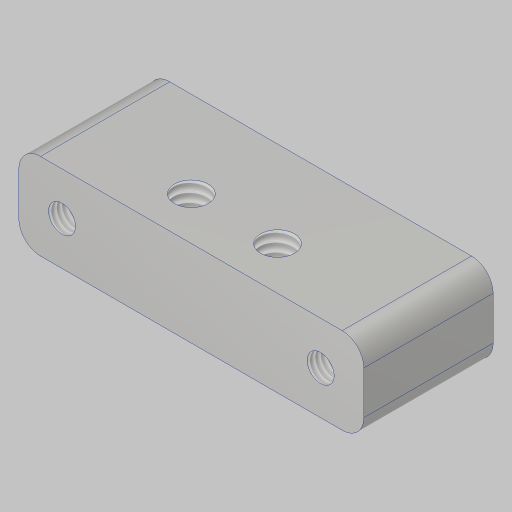
# Autodesk Inventor part: CL7-014
Saved by Autodesk Inventor 2023.5 (Build 275446000, 446)
## iProperties
Created: 2025-03-18
Part Number: CL7-014
Material: Aluminum 6061
Document SubType Name: Modeling
Designer: slick
Density: 2.7 g/cm^3
Appearance: Aluminum - Flat
Author: slick
Autodesk Inventor part; units mm, degrees
ref_plane "YZ Plane" through (0, 0, 0) normal (1, 0, 0) x (0, 1, 0)
ref_plane "XZ Plane" through (0, 0, 0) normal (0, 1, 0) x (-1, 0, 0)
ref_plane "XY Plane" through (0, 0, 0) normal (0, 0, 1) x (1, 0, 0)
sketch "Sketch1" plane through (0, 0, 0) normal (0, 0, 1) x (1, 0, 0)
  line L0 (25.4, -6.35) -> (-25.4, -6.35)
  line L1 (-25.4, -6.35) -> (-25.4, 6.35)
  line L2 (-25.4, 6.35) -> (25.4, 6.35)
  line L3 (25.4, 6.35) -> (25.4, -6.35)
  line L4 (25.4, -6.35) -> (-25.4, 6.35) construction
  line L5 (-25.4, -6.35) -> (25.4, 6.35) construction
  point P0 (0, 0)
  dimension "d0" = 50.8
  dimension "d1" = 12.7
  constraints: 12 end point, 2 midpoint, 2 parallel, 1 horizontal, 1 perpendicular
  measures "d0" distance of L1.end L2.end
  measures "d1" distance of L0.end L1.end
extrude "Extrusion1" add sketch "Sketch1" along normal blind 19.05
sketch "Sketch2" plane through (-25.4, 6.35, 0) normal (0, 1, 0) x (1, 0, 0)
  line L0 (0, 0) -> (0, -19.05) construction
  line L1 (19.05, -12.7) -> (31.75, -12.7) construction
  line L2 (50.8, 0) -> (0, 0) construction
  line L3 (50.8, -19.05) -> (0, -19.05) construction
  point P0 (25.4, 0)
  point P1 (0, -9.525)
  point P2 (25.4, -12.7)
  point P3 (25.4, 0)
  point P4 (25.4, 0)
  dimension "d4" = 12.7
  dimension "d20" = 6.35
  constraints: 4 midpoint, 2 end point, 2 vertical alignment, 1 horizontal alignment
  measures "d4" distance of L1.start L1.end
  measures "d20" distance between parallel lines of L3 L1
hole "Hole1" at (-6.35, 6.35, 12.7) at (6.35, 6.35, 12.7) direction (0, -1, 0) diameter 4.9784 end through all thread size "1/4-20 UNC" class "2B" standard "ANSI Unified Screw Threads"
sketch "Sketch3" plane through (0, 0, 19.05) normal (0, 0, 1) x (1, 0, 0)
  line L0 (-19.05, 0) -> (19.05, 0) construction
  line L1 (-25.4, 6.35) -> (-25.4, -6.35) construction
  line L2 (25.4, 6.35) -> (-25.4, 6.35) construction
  point P0 (0, 0)
  point P1 (-25.4, 0)
  point P2 (0, 0)
  point P3 (0, 6.35)
  dimension "d12" = 38.1
  constraints: 3 midpoint, 2 end point, 1 horizontal, 1 horizontal alignment, 1 vertical alignment
  measures "d12" distance of L0.start L0.end
hole "Hole2" at (-19.05, 0, 19.05) at (19.05, 0, 19.05) direction (0, 0, -1) diameter 3.9624 end through all thread size "10-32 UNF" class "2B" standard "ANSI Unified Screw Threads"
fillet "Fillet1" radius 3.175 4 edges at (-25.4, 6.35, 9.525) (-25.4, -6.35, 9.525) (25.4, 6.35, 9.525) (25.4, -6.35, 9.525)
body "Solid1"
